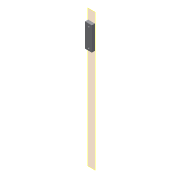
# Autodesk Inventor part: 16_Opentrons_Microscope_Slide_Bearing
Saved by Autodesk Inventor 2019.4 (Build 234330000, 330)
## iProperties
Created: 2021-01-13
Part Number: 16_Opentrons_Microscope_Slide_Bearing
Material: Generic
Document SubType Name: Modeling
Designer: diederichbenedict
Density: 1 g/cm^3
Appearance: Default
Author: diederichbenedict
Autodesk Inventor part; units mm, degrees
ref_plane "YZ Plane" through (0, 0, 0) normal (1, 0, 0) x (0, 1, 0)
ref_plane "XZ Plane" through (0, 0, 0) normal (0, 1, 0) x (-1, 0, 0)
ref_plane "XY Plane" through (0, 0, 0) normal (0, 0, 1) x (1, 0, 0)
ref_plane "Work Plane1" through (0, 0, 0) normal (0, 0, 1) x (1, 0, 0)
sketch "Sketch1" plane through (0, 0, 0) normal (0, 0, 1) x (1, 0, 0)
  line L0 (0, -200) -> (10.9676, -200) projected
  line L1 (10.9676, 0) -> (10.9676, -200) projected
  line L2 (0, 0) -> (10.9676, 0) projected
  line L3 (0, 0) -> (0, -200) projected
  circle A0 centre (5.4838, -10) radius 3 projected
  circle A1 centre (5.4838, -65) radius 3 projected
  circle A2 centre (5.4838, -40) radius 3 projected
  circle A3 centre (5.4838, -90) radius 3 projected
  circle A4 centre (5.4838, -115) radius 3 projected
  circle A5 centre (5.4838, -140) radius 3 projected
  circle A6 centre (5.4838, -165) radius 3 projected
  circle A7 centre (5.4838, -190) radius 3 projected
  line L4 (-130.7355, -19.8691) -> (119.2645, -19.8691)
  line L5 (-130.7355, -25.8691) -> (119.2645, -25.8691)
  line L6 (0, -44) -> (10.9676, -44)
  line L7 (10.9676, -44) -> (10.9676, -6)
  line L8 (10.9676, -6) -> (0, -6)
  line L9 (0, -6) -> (0, -44)
  circle A8 centre (5.4838, -40) radius 1.45
  circle A9 centre (5.4838, -10) radius 1.45
  dimension "d0" = 4
  dimension "d1" = 4
  dimension "d2" = 2.9
  dimension "d3" = 2.9
  constraints: 12 end point, 3 horizontal, 2 centre point, 2 coincident, 2 parallel, 2 point on line, 1 perpendicular, 4 other
  measures "d0" distance from line of A0.centre L8
  measures "d1" distance from line of A2.centre L6
  measures "d2" diameter of A8
  measures "d3" diameter of A9
extrude "Extrusion1" add sketch "Sketch1" along normal blind 5 contours L3 L5 L1 L6 | L3 L4 L1 L5 | L3 L8 L1 L4 | A0 | A2
sketch "Sketch2" plane through (0, 0, 5) normal (0, 0, 1) x (1, 0, 0)
  line L0 (-130.7355, -19.8691) -> (119.2645, -19.8691)
  line L1 (-130.7355, -25.8691) -> (119.2645, -25.8691)
  circle A0 centre (5.4838, -40) radius 1.45 projected
  circle A1 centre (5.4838, -10) radius 1.45 projected
  line L2 (10.9676, -44) -> (10.9676, -6) projected
  line L3 (10.9676, -6) -> (0, -6) projected
  line L4 (0, -6) -> (0, -44) projected
  line L5 (0, -44) -> (10.9676, -44) projected
  circle A2 centre (5.4838, -19.3691) radius 2.45
  circle A3 centre (5.4838, -26.3691) radius 2.45
  line L6 (10.9676, -44) -> (10.9676, -6) projected
  point P0 (0, 0)
  dimension "d6" = 4.9
  dimension "d7" = 4.9
  dimension "d8" = 0.5
  dimension "d10" = 0.5
  constraints: 4 end point, 2 centre point, 2 horizontal, 4 other
  measures "d6" diameter of A2
  measures "d7" diameter of A3
  measures "d8" distance from line of A2.centre L0
  measures "d10" distance from line of A3.centre L1
extrude "Extrusion2" cut sketch "Sketch2" against normal blind 3 contours A2 L0 | L0 A2 | A3 L1 | L1 A3
body "Solid1"
